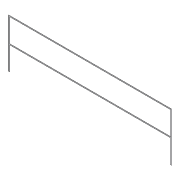
# Autodesk Inventor part: FE-00034-05
Saved by Autodesk Inventor 2012 (Build 160160000, 160)
## iProperties
Created: 2008-12-23
Part Number: FE-00034-05
Document SubType Name: Modeling
Designer: dfoster
Density: 1 g/cm^3
Material: Default
Author: dfoster
Autodesk Inventor part; units mm, degrees
ref_plane "YZ Plane" through (0, 0, 0) normal (1, 0, 0) x (0, 1, 0)
ref_plane "XZ Plane" through (0, 0, 0) normal (0, 1, 0) x (-1, 0, 0)
ref_plane "XY Plane" through (0, 0, 0) normal (0, 0, 1) x (1, 0, 0)
sketch "Sketch1" plane through (0, 0, 0) normal (0, 0, 1) x (1, 0, 0)
  line L0 (-2991.2641, -717.8588) -> (-2991.2641, 1720.5412)
  line L1 (-2991.2641, 1720.5412) -> (5155.7859, 1720.5412)
  line L2 (5155.7859, 1720.5412) -> (5155.7859, -717.8588)
  line L3 (5155.7859, -717.8588) -> (5104.9859, -717.8588)
  line L4 (5104.9859, -717.8588) -> (5104.9859, 1669.7412)
  line L5 (5104.9859, 1669.7412) -> (-2940.4641, 1669.7412)
  line L6 (-2940.4641, 1669.7412) -> (-2940.4641, -717.8588)
  line L7 (-2940.4641, -717.8588) -> (-2991.2641, -717.8588)
  line L8 (-2940.4641, 501.3412) -> (5104.9859, 501.3412)
  line L9 (5104.9859, 501.3412) -> (5104.9859, 450.5412)
  line L10 (5104.9859, 450.5412) -> (-2940.4641, 450.5412)
  line L11 (-2940.4641, 450.5412) -> (-2940.4641, 501.3412)
  dimension "d0" = 50.8
  dimension "d1" = 50.8
  dimension "d4" = 2438.4
  dimension "d14" = 1219.2
  dimension "d15" = 8147.05
  dimension "d16" = 50.8
  constraints: 24 end point, 8 parallel, 3 perpendicular, 2 collinear, 1 horizontal, 1 vertical
  measures "d0" distance between parallel lines of L5 L1
  measures "d1" distance between parallel lines of L0 L6
  measures "d4" distance of L0.start L0.end
  measures "d14" distance between parallel lines of L8 L7
  measures "d15" distance of L0.end L1.end
  measures "d16" distance between parallel lines of L2 L4
extrude "Extrusion1" add sketch "Sketch1" along normal blind 6.35 contours L0 L1 L2 L3 L4 L5 L6 L7
extrude "Extrusion3" add sketch "Sketch1" along normal blind 6.35 contours L6 L8 L4 L10
body "Solid1"
